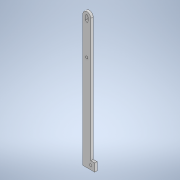
# Autodesk Inventor part: пиналка_1
Saved by Autodesk Inventor 2020 (Build 240168000, 168)
## iProperties
Created: 2025-01-29
Part Number: пиналка_1
Material: Типовые
Document SubType Name: Modeling
Designer: frozj
Density: 1 g/cm^3
Appearance: По умолчанию
Author: frozj
Autodesk Inventor part; units mm, degrees
ref_plane "YZ Plane" through (0, 0, 0) normal (1, 0, 0) x (0, 1, 0)
ref_plane "XZ Plane" through (0, 0, 0) normal (0, 1, 0) x (-1, 0, 0)
ref_plane "XY Plane" through (0, 0, 0) normal (0, 0, 1) x (1, 0, 0)
sketch "Эскиз1" plane through (0, 0, 0) normal (0, 0, 1) x (1, 0, 0)
  line L0 (-5, -82.5) -> (5, -82.5)
  line L1 (5, -82.5) -> (5, 82.5)
  line L2 (5, 82.5) -> (-5, 82.5)
  line L3 (-5, 82.5) -> (-5, -82.5)
  line L4 (-5, -82.5) -> (5, 82.5) construction
  line L5 (5, -82.5) -> (-5, 82.5) construction
  line L6 (-5, 82.5) -> (0, 82.5)
  line L7 (0, 82.5) -> (0, 77.5)
  line L8 (0, 77.5) -> (-5, 77.5)
  line L9 (-5, 77.5) -> (-5, 82.5)
  circle A0 centre (0, 77.5) radius 1.5
  line L10 (-5, 82.5) -> (5, 82.5)
  line L11 (5, 82.5) -> (5, 87.5)
  line L12 (5, 87.5) -> (-5, 87.5)
  line L13 (-5, 87.5) -> (-5, 82.5)
  circle A1 centre (0, 82.5) radius 1.5
  line L14 (-1.5, 82.5) -> (-1.5, 77.5)
  line L15 (1.5, 77.5) -> (1.5, 82.5)
  arc A2 (5, 82.5) -> (-5, 82.5) centre (0, 82.5) ccw
  line L16 (0, 77.5) -> (-5, 77.5)
  line L17 (-5, 77.5) -> (-5, 37.5)
  line L18 (-5, 37.5) -> (0, 37.5)
  line L19 (0, 37.5) -> (0, 77.5)
  circle A3 centre (0, 37.5) radius 1.5
  line L20 (-5, -82.5) -> (0, -82.5)
  line L21 (0, -82.5) -> (0, -77.5)
  line L22 (0, -77.5) -> (-5, -77.5)
  line L23 (-5, -77.5) -> (-5, -82.5)
  line L24 (-5, -82.5) -> (10, -82.5)
  line L25 (10, -82.5) -> (10, -72.5)
  line L26 (10, -72.5) -> (-5, -72.5)
  line L27 (-5, -72.5) -> (-5, -82.5)
  circle A4 centre (5, -77.5) radius 1.5
  point P0 (0, 0)
  point P1 (5, -72.5)
  dimension "d0" = 10
  dimension "d1" = 165
  dimension "d2" = 5
  dimension "d3" = 3
  dimension "d4" = 5
  dimension "d5" = 3
  dimension "d6" = 40
  dimension "d7" = 3
  dimension "d8" = 5
  dimension "d12" = 15
  dimension "d13" = 10
  dimension "d14" = 3
  constraints: 56 end point, 12 parallel, 7 perpendicular, 6 horizontal, 6 point on circle, 5 centre point, 4 coincident, 4 point on line, 2 midpoint, 1 tangent
  measures "d0" distance of L2.end L1.end
  measures "d1" distance of L1.end L0.end
  measures "d2" distance of L6.end L7.end
  measures "d3" diameter of A0
  measures "d4" distance of L11.end L10.end
  measures "d5" diameter of A1
  measures "d6" distance of L17.end L16.end
  measures "d7" diameter of A3
  measures "d8" distance of L21.end L20.end
  measures "d12" distance of L26.end L25.end
  measures "d13" distance of L25.end L24.end
  measures "d14" diameter of A4
extrude "Выдавливание1" add sketch "Эскиз1" along normal blind 3 contours L3 L22 L21 L0 | L21 L22 L3 L26 L1 A4 L0 | L1 A4 L26 L25 L24 | L3 L18 A3 L19 A0 L15 L2 L1 L26 | L3 L8 A0 L19 A3 L18 | L3 L2 L14 L8 | L2 A1 A2
